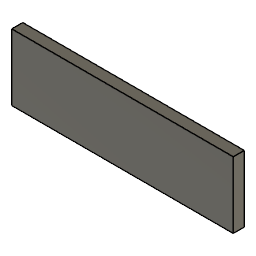
DD-fixation-v5 (Autodesk Fusion 360 design; units mm, degrees)
part number: 2025-12-22-09-38-26-040
Autodesk Fusion 360 part; units mm, degrees
sketch "Esquisse1" plane through (0, 0, 0) normal (0, 1, 0) x (1, 0, 0)
  line L0 (-10, 6) -> (30, 6)
  line L1 (30, 6) -> (30, -6)
  line L2 (30, -6) -> (-10, -6)
  line L3 (-10, -6) -> (-10, 6)
  constraint horizontal L0
  constraint vertical L1
  constraint horizontal L2
  constraint vertical L3
extrude "Extrusion1" add sketch "Esquisse1" along normal blind 2
